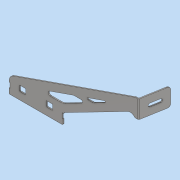
# Autodesk Inventor part: 0 零件
Saved by Autodesk Inventor 2020 (Build 240168000, 168)
## iProperties
Created: 2020-11-03
Part Number: 0 零件
Material: 不鏽鋼SUS-HL(砂紋)
Document SubType Name: Sheet Metal
Designer: p2013
Density: 8 g/cm^3
Appearance: 不鏽鋼 - 疏刷
Sheet Metal Rule: 預設 mm (_M)
Flat Pattern Width: 7.87536 cm
Flat Pattern Length: 40.0821 cm
Flat Pattern Area: 315.661 cm^2
Sheet Metal Width: 78.754 mm
Sheet Metal Length: 400.821 mm
Sheet Metal Area: 31566.113 mm^2
Author: p2013
Autodesk Inventor part; units mm, degrees
ref_plane "YZ Plane" through (0, 0, 0) normal (1, 0, 0) x (0, 1, 0)
ref_plane "XZ Plane" through (0, 0, 0) normal (0, 1, 0) x (-1, 0, 0)
ref_plane "XY Plane" through (0, 0, 0) normal (0, 0, 1) x (1, 0, 0)
sketch "草圖1" plane through (0, 0, 0) normal (0, 0, 1) x (1, 0, 0)
  line L0 (0, 0) -> (-7.8042, 0) construction
  line L1 (0, 0) -> (0, -16.694) construction
  line L2 (0, 2) -> (0, 12.5)
  line L3 (310, 145) -> (310, 102)
  line L4 (130, 19.7875) -> (130, 12.5) construction
  line L5 (128, 0) -> (2, 0)
  line L6 (310, 145) -> (368, 145)
  line L7 (375, 138) -> (375, 109)
  line L8 (368, 102) -> (310, 102)
  line L9 (332, 127.5) -> (354, 127.5)
  arc A0 (354, 119.5) -> (354, 127.5) centre (354, 123.5) ccw
  line L10 (354, 119.5) -> (332, 119.5)
  arc A1 (332, 127.5) -> (332, 119.5) centre (332, 123.5) ccw
  line L11 (65, 14) -> (65, 14) construction
  arc A2 (10.0615, 42.1637) -> (0, 28) centre (15, 28) ccw
  line L12 (10.0615, 42.1637) -> (303.401, 144.4425)
  line L13 (306.6934, 145) -> (310, 145)
  line L14 (310, 102) -> (305, 102)
  line L15 (286.6386, 106.4667) -> (135.4256, 28.6799)
  arc A3 (375, 138) -> (368, 145) centre (368, 138) ccw
  arc A4 (368, 102) -> (375, 109) centre (368, 109) ccw
  arc A5 (302.6723, 103.1075) -> (305, 102) centre (305, 105) ccw
  arc A6 (302.6723, 103.1075) -> (286.6386, 106.4667) centre (292.5854, 94.9066) ccw
  arc A7 (306.6934, 145) -> (303.401, 144.4425) centre (306.6934, 135) ccw
  arc A8 (135.4256, 28.6799) -> (131.18, 24.5) centre (140, 19.7875) ccw
  line L16 (25.9, 31) -> (39.1, 31)
  line L17 (40.1, 30) -> (40.1, 19)
  line L18 (39.1, 18) -> (25.9, 18)
  line L19 (24.9, 19) -> (24.9, 30)
  line L20 (90.9, 31) -> (104.1, 31)
  line L21 (105.1, 30) -> (105.1, 19)
  line L22 (104.1, 18) -> (90.9, 18)
  line L23 (89.9, 19) -> (89.9, 30)
  line L24 (40.1, 24.5) -> (89.9, 24.5) construction
  line L25 (0, 24.5) -> (2, 24.5)
  line L26 (2, 24.5) -> (2, 12.5)
  line L27 (2, 12.5) -> (0, 12.5)
  line L28 (0, 12.5) -> (0, 24.5) construction
  line L29 (65, 0) -> (65, 24.5) construction
  line L30 (131.18, 24.5) -> (128, 24.5)
  line L31 (128, 24.5) -> (128, 12.5)
  line L32 (128, 12.5) -> (130, 12.5)
  line L33 (130, 12.5) -> (130, 19.7875) construction
  arc A9 (0, 2) -> (2, 0) centre (2, 2) ccw
  arc A10 (128, 0) -> (130, 2) centre (128, 2) ccw
  line L34 (0, 12.5) -> (0, 24.5) construction
  line L35 (0, 24.5) -> (0, 28)
  line L36 (130, 19.7875) -> (130, 24.5) construction
  line L37 (130, 12.5) -> (130, 2)
  line L38 (123.9345, 45) -> (99.3585, 45)
  line L39 (157.566, 75) -> (173.8509, 75)
  line L40 (97.7123, 54.7212) -> (154.2737, 74.4425)
  line L41 (175.452, 68.3877) -> (135.3705, 47.769)
  arc A11 (175.452, 68.3877) -> (173.8509, 75) centre (173.8509, 71.5) ccw
  arc A12 (97.7123, 54.7212) -> (99.3585, 45) centre (99.3585, 50) ccw
  arc A13 (123.9345, 45) -> (135.3705, 47.769) centre (123.9345, 70) ccw
  arc A14 (157.566, 75) -> (154.2737, 74.4425) centre (157.566, 65) ccw
  line L42 (189.9693, 86.8885) -> (229.5263, 100.6808)
  line L43 (231.0996, 97.0139) -> (206.0106, 84.1076)
  line L44 (201.4362, 83) -> (190.6278, 83)
  arc A15 (231.0996, 97.0139) -> (229.5263, 100.6808) centre (230.1847, 98.7923) ccw
  arc A16 (201.4362, 83) -> (206.0106, 84.1076) centre (201.4362, 93) ccw
  arc A17 (189.9693, 86.8885) -> (190.6278, 83) centre (190.6278, 85) ccw
  arc A18 (24.9, 19) -> (25.9, 18) centre (25.9, 19) ccw
  arc A19 (39.1, 18) -> (40.1, 19) centre (39.1, 19) ccw
  arc A20 (40.1, 30) -> (39.1, 31) centre (39.1, 30) ccw
  arc A21 (25.9, 31) -> (24.9, 30) centre (25.9, 30) ccw
  arc A22 (90.9, 31) -> (89.9, 30) centre (90.9, 30) ccw
  arc A23 (105.1, 30) -> (104.1, 31) centre (104.1, 30) ccw
  arc A24 (104.1, 18) -> (105.1, 19) centre (104.1, 19) ccw
  arc A25 (89.9, 19) -> (90.9, 18) centre (90.9, 19) ccw
  arc A26 (131.18, 24.5) -> (130, 19.7875) centre (140, 19.7875) ccw construction
  point P0 (130, 0)
  point P1 (375, 145)
  point P2 (375, 102)
  point P3 (130, 25.8889)
  point P4 (305, 145)
  point P5 (305, 102)
  point P6 (305, 115.9121)
  point P7 (24.9, 31)
  point P8 (40.1, 18)
  point P9 (40.1, 31)
  point P10 (24.9, 18)
  point P11 (89.9, 31)
  point P12 (105.1, 18)
  point P13 (105.1, 31)
  point P14 (89.9, 18)
  point P15 (32.5, 31)
  point P16 (97.5, 31)
  point P17 (0, 10.2)
  point P18 (130, 28)
  point P19 (130, 10.2)
  dimension "d0" = 130
  dimension "d1" = 145
  dimension "d2" = 43
  dimension "d3" = 65
  dimension "d4" = 8
  dimension "d5" = 30
  dimension "d7" = 18
  dimension "d8" = 310
  dimension "d14" = 14
  dimension "d17" = 21.5
  dimension "d20" = 15
  dimension "d21" = 28
  dimension "d23" = 5
  dimension "d24" = 7
  dimension "d26" = 3
  dimension "d29" = 13
  dimension "d30" = 5
  dimension "d31" = 10
  dimension "d32" = 10
  dimension "d33" = 8
  dimension "d34" = 15.2
  dimension "d35" = 15.2
  dimension "d36" = 13
  dimension "d37" = 65
  dimension "d39" = 12
  dimension "d40" = 2
  dimension "d41" = 12.5
  dimension "d42" = 2
  dimension "d45" = 45
  dimension "d46" = 17
  dimension "d47" = 17
  dimension "d48" = 30
  dimension "d49" = 3.5
  dimension "d50" = 5
  dimension "d51" = 25
  dimension "d52" = 10
  dimension "d53" = 8
  dimension "d54" = 2
  dimension "d55" = 10
  dimension "d56" = 2
  dimension "d57" = 19.7875
  dimension "d58" = 1
  dimension "d59" = 18
  constraints: 91 end point, 60 tangent, 55 point on circle, 32 point on line, 27 centre point, 21 parallel, 11 horizontal, 9 equal radius, 7 midpoint, 7 perpendicular, 5 symmetric about line, 5 vertical, 5 vertical alignment, 4 collinear, 1 coincident
  measures "d0" distance between parallel lines of L4 L2
  measures "d1" distance from line of L3.start L5
  measures "d2" distance between parallel lines of L6 L8
  measures "d3" distance between parallel lines of L7 L3
  measures "d4" distance between parallel lines of L10 L9
  measures "d7" distance edge to line of A1 L3
  measures "d8" distance between parallel lines of L3 L2
  measures "d14" distance from line of L5 L11.start
  measures "d17" distance from line of L6 A0.centre
  measures "d20" radius of A2
  measures "d21" distance of L0.start L35.end
  measures "d23" distance of point (305, 145) L3.start
  measures "d24" radius of A3
  measures "d26" radius of A5
  measures "d29" radius of A6
  measures "d30" distance of L3.end L14.end
  measures "d31" radius of A7
  measures "d32" radius of A8
  measures "d33" angle of L15 L12
  measures "d34" distance between parallel lines of L17 L19
  measures "d35" distance between parallel lines of L21 L23
  measures "d36" distance between parallel lines of L16 L18
  measures "d37" distance of point (32.5, 31) point (97.5, 31)
  measures "d39" distance between parallel lines of L27 L25
  measures "d40" distance between parallel lines of L28 L26
  measures "d41" distance between parallel lines of L27 L5
  measures "d42" radius of A9
  measures "d45" distance between parallel lines of L5 L38
  measures "d46" distance between parallel lines of L12 L40
  measures "d47" distance between parallel lines of L15 L41
  measures "d48" distance between parallel lines of L38 L39
  measures "d49" radius of A11
  measures "d50" radius of A12
  measures "d51" radius of A13
  measures "d52" radius of A14
  measures "d53" distance between parallel lines of L39 L44
  measures "d54" radius of A15
  measures "d55" radius of A16
  measures "d56" radius of A17
  measures "d57" distance from line of A8.centre L5
  measures "d58" radius of A18
  measures "d59" distance between parallel lines of L5 L18
extrude "擠出1" add sketch "草圖1" along normal blind 2.5
bend part "折彎零件1" radius 0.5 angle 80 line through (310, 145, 0) along (0, -1, 0) centre toward (0, 0, -1) moving side (1, 0, 0) both sides no
ref_plane "工作平面1" through (65, 2, 0) normal (-1, 0, 0) x (0, 0, 1)
